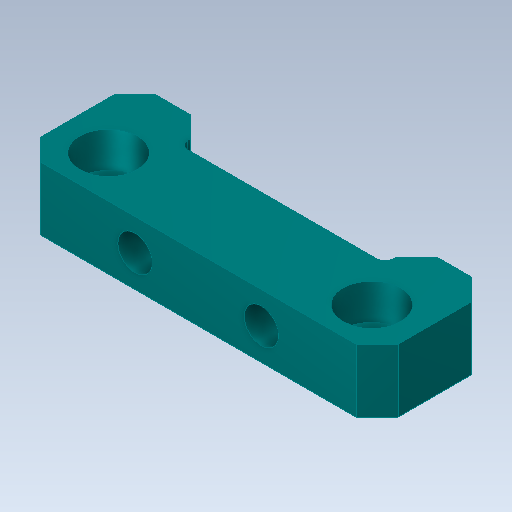
# Autodesk Inventor part: FAB-OX002x-PiezoPusherBaseComponent
Saved by Autodesk Inventor 2020 (Build 240168000, 168)
## iProperties
Created: 2017-02-10
Part Number: FAB-OX002x-PiezoPusherBaseComponent
Material: Aluminum 6061
Document SubType Name: Modeling
Designer: map
Density: 2.7 g/cm^3
Appearance: Anodized - Light Gray
shaftSeparation: 24.000 mm
Author: map
Revision Number: 01
Autodesk Inventor part; units mm, degrees
ref_plane "YZ Plane" through (0, 0, 0) normal (1, 0, 0) x (0, 1, 0)
ref_plane "XZ Plane" through (0, 0, 0) normal (0, 1, 0) x (-1, 0, 0)
ref_plane "XY Plane" through (0, 0, 0) normal (0, 0, 1) x (1, 0, 0)
sketch "Sketch1" plane through (0, 0, 0) normal (0, 1, 0) x (-1, 0, 0)
  line L0 (40.6019, 0) -> (-40.6019, 0) construction
  line L1 (0, 14.7427) -> (0, -14.7427) construction
  line L2 (25, 5) -> (-25, 5) construction
  line L3 (-25, 5) -> (-25, -5) construction
  line L4 (-25, -5) -> (25, -5) construction
  line L5 (25, -5) -> (25, 5) construction
  line L6 (34, 13) -> (-34, 13)
  line L7 (-34, 13) -> (-34, -9)
  line L8 (-34, -9) -> (34, -9)
  line L9 (34, -9) -> (34, 13)
  line L10 (26, -5) -> (24, -5) construction
  line L11 (26, -3) -> (24, -3)
  line L12 (24, -7) -> (26, -7)
  arc A0 (26, -7) -> (26, -3) centre (26, -5) ccw
  arc A1 (24, -3) -> (24, -7) centre (24, -5) ccw
  point P0 (0, 0)
  point P1 (0, 0)
  point P2 (-25, 5)
  dimension "d2" = 50
  dimension "d3" = 10
  dimension "d4" = 68
  dimension "d5" = 22
  dimension "d16" = 8
  dimension "d17" = 1
  dimension "d18" = 4
  constraints: 28 end point, 5 parallel, 4 point on circle, 4 tangent, 3 coincident, 3 horizontal, 3 midpoint, 2 centre point, 2 perpendicular, 1 point on line, 1 vertical, 3 other
  measures "d2" distance of L4.end L3.end
  measures "d3" distance of L3.end L2.end
  measures "d4" distance of L8.end L7.end
  measures "d5" distance of L7.end L6.end
  measures "d16" distance between parallel lines of L6 L2
  measures "d17" distance of L4.end L10.end
  measures "d18" diameter of A1
extrude "Extrusion1" add sketch "Sketch1" against normal blind 12 contours L9 L8 L7 L6 | A0 L12 A1 L11
sketch "Sketch6" plane through (0, -12, 0) normal (0, -1, 0) x (1, 0, 0)
  line L0 (-26, -3) -> (-24, -3) projected
  arc A0 (-26, -3) -> (-26, -7) centre (-26, -5) ccw projected
  line L1 (-24, -7) -> (-26, -7) projected
  arc A1 (-24, -7) -> (-24, -3) centre (-24, -5) ccw projected
  point P0 (0, 0)
  point P1 (25, -5)
hole "Hole5" at (25, -12, -5) direction (0, 1, 0) diameter 4 depth 8 tip angle 118
extrude "Extrusion4" cut sketch "Sketch6" against normal blind 8
hole "Hole1" at (-25, 0, 5) at (25, 0, 5) direction (0, -1, 0) diameter 6.6 end through all counterbore diameter 11 counterbore depth 6.8 clearance for "Socket Head Cap Screw ISO 4762" size "M6" standard "ISO"
sketch "Sketch3" plane through (0, 0, 0) normal (0, 1, 0) x (1, 0, 0)
  line L0 (19.5, 9) -> (-19.5, 9)
  line L1 (-19.5, 9) -> (-19.5, 3)
  line L2 (-19.5, 3) -> (19.5, 3)
  line L3 (19.5, 3) -> (19.5, 9)
  line L4 (34, 9) -> (-34, 9) projected
  line L5 (0, 0) -> (0, 9) construction
  dimension "d34" = 39
  dimension "d35" = 6
  constraints: 10 end point, 2 parallel, 1 collinear, 1 horizontal, 1 midpoint, 1 perpendicular, 1 other
  measures "d34" distance of L2.end L1.end
  measures "d35" distance of L1.end L0.end
extrude "Extrusion2" cut sketch "Sketch3" against normal through all
chamfer "Chamfer2" distance 4 angle 45 6 edges at (34, -6, -9) (34, -6, 13) (-34, -6, 13) (-34, -6, -9) (19.5, -6, -9) (-19.5, -6, -9)
fillet "Fillet2" radius 1.5 2 edges at (-19.5, -6, -3) (19.5, -6, -3)
sketch "Sketch7" plane through (18, 0, -3) normal (0, 0, -1) x (-1, 0, 0)
  line L0 (18, 0) -> (18, -12)
  line L1 (-12, -12) -> (48, -12) projected
  line L2 (30, -6) -> (6, -6)
  point P0 (18, -6)
  dimension "d67" = 24
  constraints: 4 end point, 3 midpoint, 2 coincident, 1 horizontal
  measures "d67" distance of L2.start L2.end
hole "Hole6" at (-12, -6, -3) at (12, -6, -3) direction (0, 0, 1) diameter 6.5 end through all counterbore diameter 9 counterbore depth 11
chamfer "Chamfer3" distance 0.5 angle 45 2 edges at (12, -10.5, -3) (-12, -10.5, -3)
equation "\"d67\" = shaftSeparation"
equation "\"shaftSeparation\" = 24"
body "Solid1"
